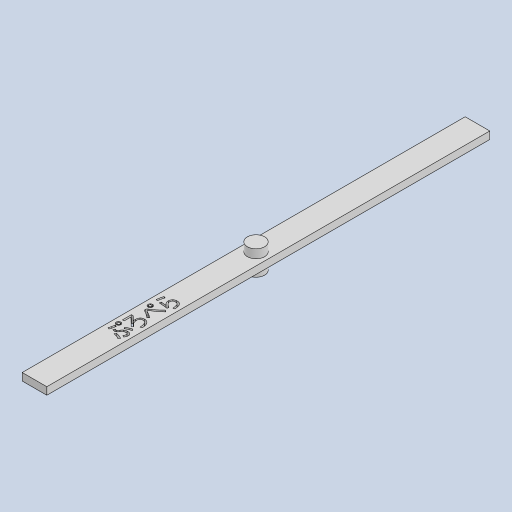
# Autodesk Inventor part: Propeller
Saved by Autodesk Inventor 2023 (Build 270158000, 158)
## iProperties
Created: 2022-06-17
Part Number: Propeller
Material: 一般
Document SubType Name: Modeling
Designer: legot
Density: 1 g/cm^3
Appearance: 既定
Author: legot
Autodesk Inventor part; units mm, degrees
ref_plane "YZ Plane" through (0, 0, 0) normal (1, 0, 0) x (0, 1, 0)
ref_plane "XZ Plane" through (0, 0, 0) normal (0, 1, 0) x (-1, 0, 0)
ref_plane "XY Plane" through (0, 0, 0) normal (0, 0, 1) x (1, 0, 0)
sketch "スケッチ1" plane through (0, 0, 0) normal (0, 1, 0) x (-1, 0, 0)
  circle A0 centre (0, 0) radius 3.5
  dimension "d0" = 7
  constraints: 1 centre point, 1 coincident
  measures "d0" diameter of A0
extrude "押し出し1" add sketch "スケッチ1" along normal mid plane 10
sketch "スケッチ2" plane through (0, 0, 0) normal (0, 1, 0) x (-1, 0, 0)
  line L0 (5, 90) -> (-5, 90)
  line L1 (-5, 90) -> (-5, -90)
  line L2 (-5, -90) -> (5, -90)
  line L3 (5, -90) -> (5, 90)
  point P0 (0, 0)
  point P1 (5, 0)
  point P2 (0, 90)
  dimension "d3" = 10
  dimension "d4" = 180
  constraints: 8 end point, 2 midpoint, 2 parallel, 1 horizontal, 1 horizontal alignment, 1 perpendicular, 1 vertical alignment
  measures "d3" distance of L0.start L0.end
  measures "d4" distance of L2.end L0.start
extrude "押し出し2" add sketch "スケッチ2" along normal mid plane 3
sketch "スケッチ3" plane through (0, 1.5, 0) normal (0, 1, 0) x (1, 0, 0)
  circle A0 centre (0, 0) radius 3.5 projected
  line L0 (-1.8414, -52.4045) -> (-1.8414, -39.4715) construction
  line L1 (-1.8414, -39.4715) -> (1.8414, -39.4715) construction
  line L2 (1.8414, -39.4715) -> (1.8414, -52.4045) construction
  line L3 (1.8414, -52.4045) -> (-1.8414, -52.4045) construction
  spline S0 degree 2 poles (-0.0173, -55.2413) (0.2101, -54.8162) (0.6402, -54.4899) knots 0 0 0 1 1 1
  spline S1 degree 2 poles (0.6402, -54.4899) (1.1295, -54.129) (1.7178, -54.0944) knots 0 0 0 1 1 1
  spline S2 degree 2 poles (1.7178, -54.0944) (2.6718, -54.0648) (3.1958, -54.4899) knots 0 0 0 1 1 1
  spline S3 degree 2 poles (3.1958, -54.4899) (3.5863, -54.8162) (3.6209, -55.3055) knots 0 0 0 1 1 1
  spline S4 degree 2 poles (3.6209, -55.3055) (3.6852, -56.1261) (3.1266, -56.9121) knots 0 0 0 1 1 1
  line L4 (3.1266, -56.9121) -> (2.4395, -56.5216)
  spline S5 degree 2 poles (2.4395, -56.5216) (2.8992, -55.7999) (2.8004, -55.2759) knots 0 0 0 1 1 1
  spline S6 degree 2 poles (2.8004, -55.2759) (2.7015, -54.7519) (1.6189, -54.8804) knots 0 0 0 1 1 1
  spline S7 degree 2 poles (1.6189, -54.8804) (0.9664, -54.9496) (0.5413, -55.6664) knots 0 0 0 1 1 1
  spline S8 degree 2 poles (0.5413, -55.6664) (-0.0173, -56.6204) (-0.5759, -56.7144) knots 0 0 0 1 1 1
  spline S9 degree 2 poles (-0.5759, -56.7144) (-0.739, -56.749) (-1.2284, -56.6501) knots 0 0 0 1 1 1
  spline S10 degree 2 poles (-1.2284, -56.6501) (-1.525, -56.5858) (-1.6881, -56.487) knots 0 0 0 1 1 1
  line L5 (-1.6881, -56.487) -> (-1.4261, -55.8345)
  spline S11 degree 2 poles (-1.4261, -55.8345) (-0.8379, -56.0273) (-0.7044, -56.0273) knots 0 0 0 1 1 1
  spline S12 degree 2 poles (-0.7044, -56.0273) (-0.4128, -55.9976) (-0.0173, -55.2413) knots 0 0 0 1 1 1
  spline S13 degree 2 poles (-3.6556, -53.2096) (-3.6852, -52.7499) (-3.3936, -52.4582) knots 0 0 0 1 1 1
  spline S14 degree 2 poles (-3.3936, -52.4582) (-3.097, -52.1962) (-2.7064, -52.1962) knots 0 0 0 1 1 1
  spline S15 degree 2 poles (-2.7064, -52.1962) (-2.2467, -52.1962) (-2.0144, -52.5225) knots 0 0 0 1 1 1
  spline S16 degree 2 poles (-2.0144, -52.5225) (-1.8216, -52.7845) (-1.787, -53.0811) knots 0 0 0 1 1 1
  spline S17 degree 2 poles (-1.787, -53.0811) (-1.7524, -53.5062) (-2.049, -53.8028) knots 0 0 0 1 1 1
  spline S18 degree 2 poles (-2.049, -53.8028) (-2.3752, -54.0944) (-2.8004, -54.0648) knots 0 0 0 1 1 1
  spline S19 degree 2 poles (-2.8004, -54.0648) (-3.1612, -54.0302) (-3.3936, -53.8028) knots 0 0 0 1 1 1
  spline S20 degree 2 poles (-3.3936, -53.8028) (-3.6556, -53.5358) (-3.6556, -53.2096) knots 0 0 0 1 1 1
  spline S21 degree 2 poles (2.5038, -58.6175) (1.5547, -57.9601) (0.0173, -57.7327) knots 0 0 0 1 1 1
  line L6 (0.0173, -57.7327) -> (0.3436, -57.0752)
  spline S22 degree 2 poles (0.3436, -57.0752) (1.7178, -57.273) (2.9635, -57.9947) knots 0 0 0 1 1 1
  line L7 (2.9635, -57.9947) -> (2.5038, -58.6175)
  spline S23 degree 2 poles (-0.1162, -53.3727) (0.8033, -52.6213) (2.2121, -52.2605) knots 0 0 0 1 1 1
  line L8 (2.2121, -52.2605) -> (2.6718, -52.9179)
  spline S24 degree 2 poles (2.6718, -52.9179) (1.2927, -53.2096) (0.309, -53.8967) knots 0 0 0 1 1 1
  line L9 (0.309, -53.8967) -> (-0.1162, -53.3727)
  spline S25 degree 2 poles (-3.359, -56.7836) (-3.1958, -56.3881) (-3.0327, -55.701) knots 0 0 0 1 1 1
  spline S26 degree 2 poles (-3.0327, -55.701) (-2.8696, -55.0139) (-2.835, -54.4207) knots 0 0 0 1 1 1
  line L10 (-2.835, -54.4207) -> (-2.1132, -54.6184)
  spline S27 degree 2 poles (-2.1132, -54.6184) (-2.2467, -55.8987) (-2.6718, -57.0456) knots 0 0 0 1 1 1
  line L11 (-2.6718, -57.0456) -> (-3.359, -56.7836)
  spline S28 degree 2 poles (-2.2467, -53.1107) (-2.2467, -52.8833) (-2.3752, -52.7845) knots 0 0 0 1 1 1
  spline S29 degree 2 poles (-2.3752, -52.7845) (-2.5087, -52.6213) (-2.7064, -52.651) knots 0 0 0 1 1 1
  spline S30 degree 2 poles (-2.7064, -52.651) (-2.8696, -52.651) (-3.0327, -52.7845) knots 0 0 0 1 1 1
  spline S31 degree 2 poles (-3.0327, -52.7845) (-3.1612, -52.8833) (-3.1958, -53.1107) knots 0 0 0 1 1 1
  spline S32 degree 2 poles (-3.1958, -53.1107) (-3.1612, -53.3085) (-3.0327, -53.4716) knots 0 0 0 1 1 1
  spline S33 degree 2 poles (-3.0327, -53.4716) (-2.8696, -53.6051) (-2.7064, -53.6051) knots 0 0 0 1 1 1
  spline S34 degree 2 poles (-2.7064, -53.6051) (-2.4741, -53.6051) (-2.3752, -53.4419) knots 0 0 0 1 1 1
  spline S35 degree 2 poles (-2.3752, -53.4419) (-2.2467, -53.2739) (-2.2467, -53.1107) knots 0 0 0 1 1 1
  spline S36 degree 2 poles (-0.7044, -48.3306) (-0.7044, -47.3815) (-0.2447, -46.8871) knots 0 0 0 1 1 1
  spline S37 degree 2 poles (-0.2447, -46.8871) (0.1804, -46.3632) (1.0307, -46.3632) knots 0 0 0 1 1 1
  spline S38 degree 2 poles (1.0307, -46.3632) (2.1132, -46.3335) (2.8004, -47.1491) knots 0 0 0 1 1 1
  spline S39 degree 2 poles (2.8004, -47.1491) (3.5567, -48.034) (3.6209, -49.8383) knots 0 0 0 1 1 1
  line L12 (3.6209, -49.8383) -> (2.9635, -50.0657)
  spline S40 degree 2 poles (2.9635, -50.0657) (2.8992, -48.4937) (2.3752, -47.7423) knots 0 0 0 1 1 1
  spline S41 degree 2 poles (2.3752, -47.7423) (1.9155, -47.0849) (1.1938, -47.0503) knots 0 0 0 1 1 1
  spline S42 degree 2 poles (1.1938, -47.0503) (0.4721, -47.0206) (0.1162, -47.4803) knots 0 0 0 1 1 1
  spline S43 degree 2 poles (0.1162, -47.4803) (-0.1162, -47.8066) (-0.1162, -48.4294) knots 0 0 0 1 1 1
  spline S44 degree 2 poles (-0.1162, -48.4294) (-0.1162, -49.3143) (0.3436, -50.036) knots 0 0 0 1 1 1
  spline S45 degree 2 poles (0.3436, -50.036) (0.6698, -50.4611) (1.4904, -51.1828) knots 0 0 0 1 1 1
  line L13 (1.4904, -51.1828) -> (0.9318, -51.6722)
  spline S46 degree 2 poles (0.9318, -51.6722) (0.0816, -50.7874) (-0.9368, -49.8383) knots 0 0 0 1 1 1
  spline S47 degree 2 poles (-0.9368, -49.8383) (-1.9501, -48.82) (-2.4444, -48.4294) knots 0 0 0 1 1 1
  line L14 (-2.4444, -48.4294) -> (-2.4444, -51.1136)
  line L15 (-2.4444, -51.1136) -> (-3.1612, -51.1136)
  line L16 (-3.1612, -51.1136) -> (-3.1612, -47.4457)
  line L17 (-3.1612, -47.4457) -> (-2.4741, -47.4457)
  spline S48 degree 2 poles (-2.4741, -47.4457) (-1.787, -48.0686) (-0.5067, -49.3439) knots 0 0 0 1 1 1
  spline S49 degree 2 poles (-0.5067, -49.3439) (-0.7044, -48.9188) (-0.7044, -48.3306) knots 0 0 0 1 1 1
  spline S50 degree 2 poles (-2.1825, -42.8238) (-2.1825, -42.3294) (-1.787, -42.1021) knots 0 0 0 1 1 1
  spline S51 degree 2 poles (-1.787, -42.1021) (0.3436, -40.8267) (2.1132, -38.9581) knots 0 0 0 1 1 1
  line L18 (2.1132, -38.9581) -> (2.8004, -39.5118)
  spline S52 degree 2 poles (2.8004, -39.5118) (0.8329, -41.3803) (-1.1641, -42.4975) knots 0 0 0 1 1 1
  spline S53 degree 2 poles (-1.1641, -42.4975) (-1.3619, -42.5964) (-1.3619, -42.7892) knots 0 0 0 1 1 1
  spline S54 degree 2 poles (-1.3619, -42.7892) (-1.3619, -42.9869) (-1.1641, -43.0858) knots 0 0 0 1 1 1
  spline S55 degree 2 poles (-1.1641, -43.0858) (-0.5759, -43.3824) (0.1458, -43.8075) knots 0 0 0 1 1 1
  spline S56 degree 2 poles (0.1458, -43.8075) (1.1938, -44.4303) (1.6535, -44.8555) knots 0 0 0 1 1 1
  line L19 (1.6535, -44.8555) -> (1.0307, -45.3794)
  spline S57 degree 2 poles (1.0307, -45.3794) (0.3436, -44.6577) (-1.6239, -43.5751) knots 0 0 0 1 1 1
  spline S58 degree 2 poles (-1.6239, -43.5751) (-1.9501, -43.3824) (-2.0836, -43.15) knots 0 0 0 1 1 1
  spline S59 degree 2 poles (-2.0836, -43.15) (-2.1825, -42.9869) (-2.1825, -42.8238) knots 0 0 0 1 1 1
  spline S60 degree 2 poles (-3.4232, -40.4658) (-3.4232, -40.0704) (-3.097, -39.7738) knots 0 0 0 1 1 1
  spline S61 degree 2 poles (-3.097, -39.7738) (-2.8696, -39.581) (-2.5384, -39.5464) knots 0 0 0 1 1 1
  spline S62 degree 2 poles (-2.5384, -39.5464) (-2.0836, -39.5118) (-1.8216, -39.8084) knots 0 0 0 1 1 1
  spline S63 degree 2 poles (-1.8216, -39.8084) (-1.5596, -40.0704) (-1.5596, -40.3966) knots 0 0 0 1 1 1
  spline S64 degree 2 poles (-1.5596, -40.3966) (-1.525, -40.8563) (-1.8216, -41.1529) knots 0 0 0 1 1 1
  spline S65 degree 2 poles (-1.8216, -41.1529) (-2.0836, -41.4149) (-2.4444, -41.4149) knots 0 0 0 1 1 1
  spline S66 degree 2 poles (-2.4444, -41.4149) (-2.835, -41.4149) (-3.1316, -41.1529) knots 0 0 0 1 1 1
  spline S67 degree 2 poles (-3.1316, -41.1529) (-3.3936, -40.8563) (-3.4232, -40.4658) knots 0 0 0 1 1 1
  spline S68 degree 2 poles (-2.0144, -40.4658) (-2.0144, -40.2681) (-2.1479, -40.1346) knots 0 0 0 1 1 1
  spline S69 degree 2 poles (-2.1479, -40.1346) (-2.2764, -40.0061) (-2.4741, -40.0061) knots 0 0 0 1 1 1
  spline S70 degree 2 poles (-2.4741, -40.0061) (-2.6076, -40.0061) (-2.7707, -40.105) knots 0 0 0 1 1 1
  spline S71 degree 2 poles (-2.7707, -40.105) (-2.9684, -40.2681) (-2.9684, -40.4658) knots 0 0 0 1 1 1
  spline S72 degree 2 poles (-2.9684, -40.4658) (-2.9684, -40.6586) (-2.835, -40.7921) knots 0 0 0 1 1 1
  spline S73 degree 2 poles (-2.835, -40.7921) (-2.6718, -40.9206) (-2.4741, -40.9552) knots 0 0 0 1 1 1
  spline S74 degree 2 poles (-2.4741, -40.9552) (-2.2467, -40.9206) (-2.1479, -40.7921) knots 0 0 0 1 1 1
  spline S75 degree 2 poles (-2.1479, -40.7921) (-2.0144, -40.629) (-2.0144, -40.4658) knots 0 0 0 1 1 1
  spline S76 degree 2 poles (-0.5413, -35.0579) (-0.5067, -34.2422) (0.0173, -33.7825) knots 0 0 0 1 1 1
  spline S77 degree 2 poles (0.0173, -33.7825) (0.4424, -33.3871) (1.1295, -33.3574) knots 0 0 0 1 1 1
  spline S78 degree 2 poles (1.1295, -33.3574) (2.4098, -33.2882) (2.9635, -34.0742) knots 0 0 0 1 1 1
  spline S79 degree 2 poles (2.9635, -34.0742) (3.4875, -34.7959) (3.6506, -36.6002) knots 0 0 0 1 1 1
  line L20 (3.6506, -36.6002) -> (2.9635, -36.7287)
  spline S80 degree 2 poles (2.9635, -36.7287) (2.8646, -35.0925) (2.4098, -34.5042) knots 0 0 0 1 1 1
  spline S81 degree 2 poles (2.4098, -34.5042) (2.1132, -34.0742) (1.3915, -34.0445) knots 0 0 0 1 1 1
  spline S82 degree 2 poles (1.3915, -34.0445) (0.7687, -34.0099) (0.4721, -34.2422) knots 0 0 0 1 1 1
  spline S83 degree 2 poles (0.4721, -34.2422) (0.0816, -34.5685) (0.047, -35.221) knots 0 0 0 1 1 1
  spline S84 degree 2 poles (0.047, -35.221) (0.047, -35.7499) (0.6402, -36.3679) knots 0 0 0 1 1 1
  spline S85 degree 2 poles (0.6402, -36.3679) (1.1641, -36.8968) (1.9155, -37.3219) knots 0 0 0 1 1 1
  line L21 (1.9155, -37.3219) -> (1.8167, -37.9744)
  spline S86 degree 2 poles (1.8167, -37.9744) (0.7687, -37.8113) (-1.6535, -37.6482) knots 0 0 0 1 1 1
  line L22 (-1.6535, -37.6482) -> (-1.5893, -36.961)
  spline S87 degree 2 poles (-1.5893, -36.961) (-0.7687, -37.0253) (0.5709, -37.1588) knots 0 0 0 1 1 1
  spline S88 degree 2 poles (0.5709, -37.1588) (0.1162, -36.7633) (-0.215, -36.3036) knots 0 0 0 1 1 1
  spline S89 degree 2 poles (-0.215, -36.3036) (-0.5413, -35.7153) (-0.5413, -35.0579) knots 0 0 0 1 1 1
  spline S90 degree 2 poles (-3.4578, -37.0896) (-3.3293, -35.7153) (-2.8992, -34.435) knots 0 0 0 1 1 1
  line L23 (-2.8992, -34.435) -> (-2.2121, -34.697)
  spline S91 degree 2 poles (-2.2121, -34.697) (-2.5087, -35.5176) (-2.835, -37.2527) knots 0 0 0 1 1 1
  line L24 (-2.835, -37.2527) -> (-3.4578, -37.0896)
  point P0 (0, -52.4045)
  constraints: 1 midpoint, 1 vertical, 1 vertical alignment, 2 other
extrude "押し出し3" cut sketch "スケッチ3" against normal through all contours S0 S1 S2 S3 S4 L4 S5 S6 S7 S8 S9 S10 L5 S11 S12 | S13 S14 S15 S16 S17 S18 S19 S20 | S21 L6 S22 L7 | S23 L8 S24 L9 | S25 S26 L10 S27 L11 | S36 S37 S38 S39 L12 S40 S41 S42 S43 S44 S45 L13 S46 S47 L14 L15 L16 L17 S48 S49 | S50 S51 L18 S52 S53 S54 S55 S56 L19 S57 S58 S59 | S60 S61 S62 S63 S64 S65 S66 S67 | S76 S77 S78 S79 L20 S80 S81 S82 S83 S84 S85 L21 S86 L22 S87 S88 S89 | S90 L23 S91 L24
